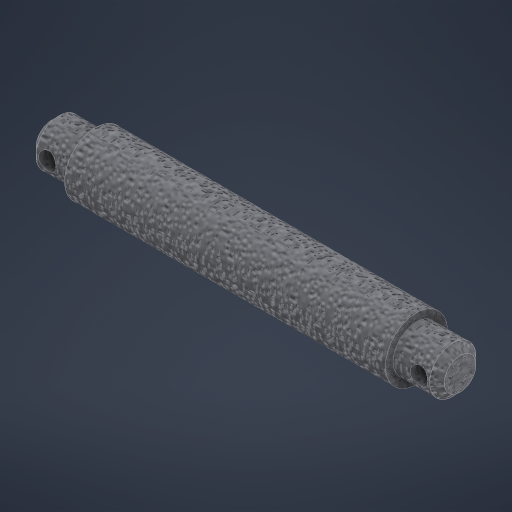
# Autodesk Inventor part: Cannon Pin
Saved by Autodesk Inventor 2024.1 (Build 281209000, 209)
## iProperties
Created: 2023-10-23
Part Number: Cannon Pin
Material: Iron, Cast
Document SubType Name: Modeling
Designer: LEGION SMIT
Density: 7.15 g/cm^3
Appearance: Iron - Cast
Author: LEGION SMIT
Autodesk Inventor part; units mm, degrees
ref_plane "YZ Plane" through (0, 0, 0) normal (1, 0, 0) x (0, 1, 0)
ref_plane "XZ Plane" through (0, 0, 0) normal (0, 1, 0) x (-1, 0, 0)
sketch "Sketch1" plane through (0, 0, 0) normal (0, 1, 0) x (-1, 0, 0)
  line L0 (0, 0) -> (0, 3.175)
  line L1 (0, 3.175) -> (-6, 3.175)
  line L2 (-6, 3.175) -> (-6, 4.25)
  line L3 (-6, 4.25) -> (-50, 4.25)
  line L4 (-50, 4.25) -> (-50, 3.175)
  line L5 (-50, 3.175) -> (-56, 3.175)
  line L6 (-56, 3.175) -> (-56, 0)
  line L7 (-56, 0) -> (0, 0)
  dimension "d0" = 56
  dimension "d1" = 6
  dimension "d2" = 6
  dimension "d3" = 4.25
  dimension "d4" = 3.175
  constraints: 16 end point, 6 perpendicular, 2 point on line, 1 vertical
  measures "d0" distance between parallel lines of L6 L0
  measures "d1" distance of L0.end L1.end
  measures "d2" distance of L4.end L5.end
  measures "d3" distance between parallel lines of L7 L3
  measures "d4" distance between parallel lines of L7 L1
revolve "Revolution1" add sketch "Sketch1" angle 360 about axis through (56, 0, 0) along (-1, 0, 0)
chamfer "Chamfer1" distance 1 angle 45 2 edges at (0, 0, -3.175) (56, 0, -3.175)
sketch "Sketch2" plane through (0, 0, 0) normal (0, 1, 0) x (-1, 0, 0)
  circle A0 centre (-2.5, 0) radius 1.2
  line L0 (0, 2.175) -> (0, -2.175) projected
  circle A1 centre (-53.5, 0) radius 1.2
  line L1 (-56, -2.175) -> (-56, 2.175) projected
  point P0 (0, 0)
  point P1 (0, 0)
  point P2 (-56, 0)
  dimension "d9" = 2.4
  dimension "d10" = 2.5
  dimension "d11" = 2.4
  dimension "d12" = 2.5
  constraints: 2 centre point, 2 horizontal alignment, 2 midpoint
  measures "d9" diameter of A0
  measures "d10" distance from line of L0 A0.centre
  measures "d11" diameter of A1
  measures "d12" distance from line of L1 A1.centre
extrude "Extrusion1" cut sketch "Sketch2" along normal mid plane 10
ref_plane "Work Plane1" through (28, 0, 0) normal (-1, 0, 0) x (0, 0, 1)
body "Solid1"
